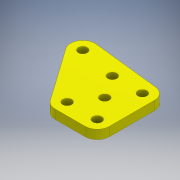
# Autodesk Inventor part: LegBase_back
Saved by Autodesk Inventor 2016 (Build 200138000, 138)
## iProperties
Created: 2015-12-07
Part Number: LegBase_back
Material: Generic
Document SubType Name: Modeling
Designer: lk8187
Density: 1 g/cm^3
Appearance: Smooth - Yellow
Author: lk8187
Autodesk Inventor part; units mm, degrees
ref_plane "YZ Plane" through (0, 0, 0) normal (1, 0, 0) x (0, 1, 0)
ref_plane "XZ Plane" through (0, 0, 0) normal (0, 1, 0) x (-1, 0, 0)
ref_plane "XY Plane" through (0, 0, 0) normal (0, 0, 1) x (1, 0, 0)
sketch "Sketch1" plane through (0, 0, 0) normal (0, 0, 1) x (1, 0, 0)
  line L0 (0, 0) -> (-17.3205, 10) construction
  line L1 (5, -7.5) -> (-5, -7.5) construction
  line L2 (-5, -7.5) -> (-5, 7.5) construction
  line L3 (-5, 7.5) -> (5, 7.5) construction
  line L4 (5, 7.5) -> (5, -7.5) construction
  line L5 (5, -7.5) -> (-5, 7.5) construction
  line L6 (-5, -7.5) -> (5, 7.5) construction
  line L7 (-16.8753, 13.9751) -> (5.4452, 11.4751)
  arc A0 (9, 7.5) -> (5.4452, 11.4751) centre (5, 7.5) ccw
  line L8 (9, 7.5) -> (9, -7.5)
  arc A1 (5, -11.5) -> (9, -7.5) centre (5, -7.5) ccw
  line L9 (5, -11.5) -> (-5, -11.5)
  arc A2 (-8.2707, -9.8027) -> (-5, -11.5) centre (-5, -7.5) ccw
  line L10 (-8.2707, -9.8027) -> (-20.5912, 7.6973)
  arc A3 (-16.8753, 13.9751) -> (-20.5912, 7.6973) centre (-17.3205, 10) ccw
  dimension "d0" = 10
  dimension "d1" = 15
  dimension "d2" = 20
  dimension "d3" = 30
  dimension "d4" = 4
  constraints: 22 end point, 10 coincident, 8 point on circle, 8 tangent, 4 centre point, 3 equal radius, 2 horizontal, 2 midpoint, 2 parallel, 1 perpendicular
  measures "d0" distance of L2.end L3.end
  measures "d1" distance of L3.end L1.start
  measures "d2" distance of L0.start L0.end
  measures "d3" angle of L3 L0
  measures "d4" radius of A0
extrude "Extrusion1" add sketch "Sketch1" against normal blind 3
hole "Hole1" at (-17.3205, 10, 0) at (-5, 7.5, 0) at (5, 7.5, 0) at (5, -7.5, 0) at (-5, -7.5, 0) direction (0, 0, -1) diameter 3 depth 8 tip angle 118
hole "Hole2" at (0, 0, 0) direction (0, 0, -1) diameter 3 depth 8 tip angle 118
body "Solid1"
